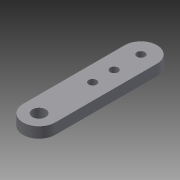
# Autodesk Inventor part: z axis arm2
Saved by Autodesk Inventor 2013 (Build 170138000, 138)
## iProperties
Created: 2017-03-09
Part Number: z axis arm2
Material: Generic
Document SubType Name: Modeling
Designer: Herman de Vries
Density: 1 g/cm^3
Author: Herman de Vries
Autodesk Inventor part; units mm, degrees
ref_plane "YZ Plane" through (0, 0, 0) normal (1, 0, 0) x (0, 1, 0)
ref_plane "XZ Plane" through (0, 0, 0) normal (0, 1, 0) x (-1, 0, 0)
ref_plane "XY Plane" through (0, 0, 0) normal (0, 0, 1) x (1, 0, 0)
sketch "Sketch1" plane through (0, 0, 0) normal (0, 0, 1) x (1, 0, 0)
  line L0 (0, 0) -> (12, 0) construction
  line L1 (12, 0) -> (12, 38)
  line L2 (12, 38) -> (0, 38) construction
  line L3 (0, 38) -> (0, 0)
  arc A0 (12, 38) -> (0, 38) centre (6, 38) ccw
  arc A1 (0, 0) -> (12, 0) centre (6, 0) ccw
  circle A2 centre (6, 38) radius 1.5
  circle A3 centre (6, 0) radius 2.5
  circle A4 centre (6, 20) radius 1.5
  circle A5 centre (6, 28) radius 1.5
  dimension "d0" = 12
  dimension "d1" = 38
  dimension "d2" = 3
  dimension "d3" = 5
  dimension "d6" = 3
  dimension "d7" = 20
  dimension "d8" = 3
  dimension "d9" = 10
  constraints: 8 end point, 6 centre point, 4 point on circle, 2 coincident, 2 midpoint, 2 parallel, 2 vertical alignment, 1 horizontal, 1 perpendicular
  measures "d0" distance of L2.end L1.end
  measures "d1" distance of L1.end L0.end
  measures "d2" diameter of A2
  measures "d3" diameter of A3
  measures "d6" diameter of A4
  measures "d7" distance of A1.centre A4.centre
  measures "d8" diameter of A5
  measures "d9" distance of A5.centre A0.centre
extrude "Extrusion1" add sketch "Sketch1" along normal blind 4
body "Solid1"
